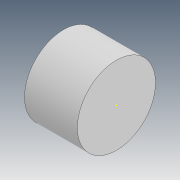
# Autodesk Inventor part: roda sup
Saved by Autodesk Inventor 2021 (Build 250183000, 183)
## iProperties
Created: 2020-10-08
Part Number: roda sup
Material: Genérico
Document SubType Name: Modeling
Designer: evert
Density: 1 g/cm^3
Appearance: Padrão
Author: evert
Autodesk Inventor part; units mm, degrees
ref_plane "YZ Plane" through (0, 0, 0) normal (1, 0, 0) x (0, 1, 0)
ref_plane "XZ Plane" through (0, 0, 0) normal (0, 1, 0) x (-1, 0, 0)
ref_plane "XY Plane" through (0, 0, 0) normal (0, 0, 1) x (1, 0, 0)
sketch "Esboço1" plane through (0, 0, 0) normal (0, 0, 1) x (1, 0, 0)
  line L0 (0, 0) -> (9, 0)
  line L1 (9, 0) -> (9, 6.65)
  line L2 (9, 6.65) -> (0, 6.65)
  line L3 (0, 6.65) -> (0, 4.65)
  line L4 (0, 4.65) -> (2.5, 4.65)
  line L5 (2.5, 4.65) -> (2.5, 0)
  dimension "d0" = 9
  dimension "d1" = 6.65
  dimension "d2" = 2
  dimension "d3" = 2.5
  constraints: 12 end point, 4 perpendicular, 2 horizontal, 1 point on line
  measures "d0" distance of L0.start L0.end
  measures "d1" distance of L0.end L1.end
  measures "d2" distance of L2.end L3.end
  measures "d3" distance of L3.end L4.end
revolve "Revolução1" add sketch "Esboço1" angle 360 about axis through (0, 0, 0) along (1, 0, 0)
sketch "Esboço2" plane through (9, 0, 0) normal (1, 0, 0) x (0, 0, -1)
  circle A0 centre (0, 0) radius 2
  dimension "d5" = 4
  constraints: 1 centre point, 1 coincident
  measures "d5" diameter of A0
extrude "Extrusão1" add sketch "Esboço2" along normal blind 1.5
sketch "Esboço3" plane through (2.5, 0, 0) normal (-1, 0, 0) x (0, 0, 1)
  circle A0 centre (0, 0) radius 1.5
  dimension "d8" = 3
  constraints: 1 centre point, 1 coincident
  measures "d8" diameter of A0
extrude "Extrusão2" cut sketch "Esboço3" against normal blind 4
sketch "Esboço4" plane through (0, 0, 0) normal (-1, 0, 0) x (0, 0, 1)
  point P0 (0, 0)
sketch "Esboço5" plane through (9, 0, 0) normal (1, 0, 0) x (0, 0, -1)
  point P0 (0, 0)
sketch "Esboço6" plane through (10.5, 0, 0) normal (1, 0, 0) x (0, 0, -1)
  circle A0 centre (0, 0) radius 2 projected
  circle A1 centre (0, 0) radius 1
  dimension "d11" = 2
  constraints: 1 centre point, 1 coincident
  measures "d11" diameter of A1
extrude "Extrusão3" cut sketch "Esboço6" against normal blind 1.06 contours A1
sketch "Esboço7" plane through (10.5, 0, 0) normal (1, 0, 0) x (0, 0, -1)
  circle A0 centre (0, 0) radius 2
  constraints: 1 centre point, 1 coincident
extrude "Extrusão4" cut sketch "Esboço7" against normal blind 1.5
